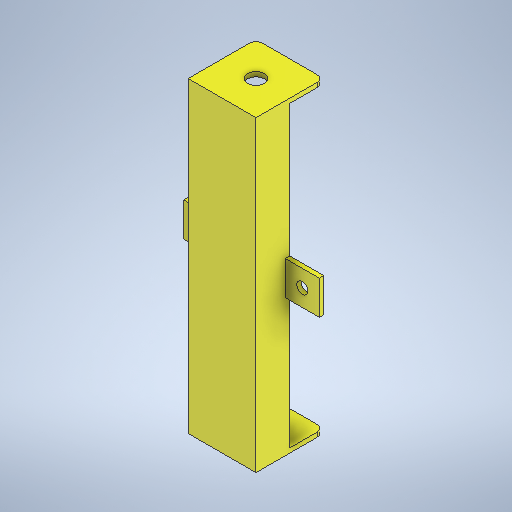
# Autodesk Inventor part: Motorhalterung_Teil1.1
Saved by Autodesk Inventor 2025.1 (Build 291241000, 241)
## iProperties
Created: 2024-12-19
Part Number: Motorhalterung_Teil1.1
Material: Generisch
Document SubType Name: Modeling
Designer: Julian
Density: 1 g/cm^3
Appearance: Vorgabe
Author: Julian
Autodesk Inventor part; units mm, degrees
ref_plane "YZ Plane" through (0, 0, 0) normal (1, 0, 0) x (0, 1, 0)
ref_plane "XZ Plane" through (0, 0, 0) normal (0, 1, 0) x (-1, 0, 0)
ref_plane "XY Plane" through (0, 0, 0) normal (0, 0, 1) x (1, 0, 0)
sketch "Skizze1" plane through (0, 0, 0) normal (0, 0, 1) x (1, 0, 0)
  line L0 (15, 7.5) -> (15, -7.5)
  line L1 (15, -7.5) -> (-15, -7.5)
  line L2 (-15, -7.5) -> (-15, 7.5)
  line L3 (-15, 7.5) -> (15, -7.5) construction
  line L4 (15, 7.5) -> (-15, -7.5) construction
  arc A0 (-13, 7.5) -> (13, 7.5) centre (0, 7.5) ccw
  line L5 (-15, 7.5) -> (-13, 7.5)
  line L6 (13, 7.5) -> (15, 7.5)
  point P0 (0, 0)
  dimension "d0" = 30
  dimension "d1" = 15
  dimension "d2" = 26
  constraints: 14 end point, 3 parallel, 2 horizontal, 2 midpoint, 2 perpendicular, 2 point on circle, 1 centre point
  measures "d0" distance of L0.end L1.end
  measures "d1" distance of L0.start L0.end
  measures "d2" diameter of A0
extrude "Extrusion1" add sketch "Skizze1" along normal blind 132
sketch "Skizze2" plane through (-15, -7.5, 0) normal (-1, 0, 0) x (0, 0, 1)
  line L0 (0, 15) -> (0, 2) projected
  line L1 (58.5, 15) -> (66, 15)
  line L2 (0, 15) -> (132, 15) projected
  line L3 (73.5, 15) -> (73.5, 13)
  line L4 (73.5, 13) -> (58.5, 13)
  line L5 (58.5, 13) -> (58.5, 15)
  line L6 (58.5, 17) -> (73.5, 13) construction
  line L7 (73.5, 17) -> (58.5, 13) construction
  line L8 (58.5, 15) -> (73.5, 15)
  point P0 (0, 7.5)
  dimension "d5" = 66
  constraints: 14 end point, 3 midpoint, 1 parallel
  measures "d5" distance of L0.start L1.end
extrude "Extrusion2" add sketch "Skizze2" along normal blind 15
sketch "Skizze3" plane through (15, -7.5, 0) normal (1, 0, 0) x (0, 0, -1)
  line L0 (-73.5, 15) -> (-73.5, 13)
  line L1 (-73.5, 13) -> (-58.5, 13)
  line L2 (-58.5, 13) -> (-58.5, 15)
  line L3 (-58.5, 17) -> (-73.5, 13) construction
  line L4 (-73.5, 17) -> (-58.5, 13) construction
  line L5 (-73.5, 15) -> (-58.5, 15)
  point P0 (0, 7.5)
  dimension "d11" = 15
  dimension "d12" = 4
  constraints: 12 end point, 1 parallel
  measures "d11" distance of L1.end L0.end
  measures "d12" distance of L0.end L4.start
extrude "Extrusion3" add sketch "Skizze3" along normal blind 15
sketch "Skizze4" plane through (13, 7.5, 132) normal (0, 1, 0) x (1, 0, 0)
  line L0 (2, 58.5) -> (17, 58.5) projected
  line L1 (2, 73.5) -> (2, 58.5) projected
  line L2 (2, 73.5) -> (17, 73.5) projected
  circle A0 centre (9.5, 66) radius 2.5
  line L3 (-28, 58.5) -> (-28, 73.5) projected
  line L4 (-28, 73.5) -> (-43, 73.5) projected
  circle A1 centre (-35.5, 66) radius 2.5
  point P0 (-13, 132)
  point P1 (-43, 58.5)
  dimension "d15" = 5
  dimension "d16" = 5
  constraints: 2 centre point
  measures "d15" diameter of A0
  measures "d16" diameter of A1
extrude "Extrusion4" cut sketch "Skizze4" against normal blind 15
sketch "Skizze5" plane through (0, 0, 0) normal (0, 0, -1) x (-1, 0, 0)
  line L0 (15, -7.5) -> (-15, -7.5) projected
  line L1 (-15, -7.5) -> (15, -7.5)
  line L2 (15, -7.5) -> (15, 22.5)
  line L3 (15, 22.5) -> (-15, 22.5)
  line L4 (-15, 22.5) -> (-15, -7.5)
  point P0 (0, 0)
  dimension "d19" = 30
  dimension "d20" = 30
  constraints: 8 end point, 2 parallel, 1 horizontal, 1 perpendicular
  measures "d19" distance of L3.end L2.end
  measures "d20" distance of L2.end L1.end
extrude "Extrusion5" add sketch "Skizze5" along normal blind 2
sketch "Skizze6" plane through (0, 0, 132) normal (0, 0, 1) x (1, 0, 0)
  line L0 (-15, -7.5) -> (15, -7.5)
  line L1 (15, -7.5) -> (15, 22.5)
  line L2 (15, 22.5) -> (-15, 22.5)
  line L3 (-15, 22.5) -> (-15, -7.5)
  point P0 (0, 0)
  dimension "d23" = 30
  dimension "d24" = 30
  constraints: 8 end point, 2 parallel, 1 horizontal, 1 perpendicular
  measures "d23" distance of L2.end L1.end
  measures "d24" distance of L1.end L0.end
extrude "Extrusion6" add sketch "Skizze6" along normal blind 2
sketch "Skizze7" plane through (0, 0, 134) normal (0, 0, 1) x (1, 0, 0)
  arc A0 (-13, 7.5) -> (13, 7.5) centre (0, 7.5) ccw projected
  circle A1 centre (0, 7.5) radius 3.75
  point P0 (0, 0)
  dimension "d27" = 7.5
  constraints: 1 centre point, 1 coincident
  measures "d27" diameter of A1
extrude "Extrusion7" cut sketch "Skizze7" against normal through all
fillet "Rundung1" radius 3 1 edges at (15, 22.5, 133)
fillet "Rundung2" radius 3 1 edges at (-15, 22.5, 133)
fillet "Rundung3" radius 3 1 edges at (-15, 22.5, -1)
fillet "Rundung4" radius 3 1 edges at (15, 22.5, -1)
